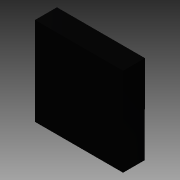
# Autodesk Inventor part: ADP1650
Saved by Autodesk Inventor 2013 (Build 170138000, 138)
## iProperties
Created: 2015-07-04
Part Number: ADP1650
Material: Ogólny
Document SubType Name: Modeling
Designer: terg
Density: 1 g/cm^3
Author: terg
Autodesk Inventor part; units mm, degrees
ref_plane "YZ Plane" through (0, 0, 0) normal (1, 0, 0) x (0, 1, 0)
ref_plane "XZ Plane" through (0, 0, 0) normal (0, 1, 0) x (-1, 0, 0)
ref_plane "XY Plane" through (0, 0, 0) normal (0, 0, 1) x (1, 0, 0)
sketch "Szkic1" plane through (0, 0, 0) normal (0, 1, 0) x (-1, 0, 0)
  line L0 (0, 0) -> (3, 0)
  line L1 (3, 0) -> (3, 3)
  line L2 (3, 3) -> (0, 3)
  line L3 (0, 3) -> (0, 0)
  dimension "d0" = 3
  dimension "d1" = 3
  constraints: 8 end point, 2 parallel, 1 horizontal, 1 perpendicular
  measures "d0" distance of L2.end L1.end
  measures "d1" distance of L1.end L0.end
extrude "Wyciągnięcie proste1" add sketch "Szkic1" along normal blind 0.75
sketch "Szkic2" plane through (0, 0.75, 0) normal (0, 1, 0) x (1, 0, 0)
  line L0 (0, 0) -> (-1.5, 0)
  line L1 (-1.5, 0) -> (-1.5, -1.5)
  line L2 (-1.5, -1.5) -> (0, -1.5)
  line L3 (0, -1.5) -> (0, 0)
  dimension "d4" = 1.5
  dimension "d5" = 1.5
  constraints: 8 end point, 2 parallel, 1 horizontal, 1 perpendicular
  measures "d4" distance of L2.end L1.end
  measures "d5" distance of L1.end L0.end
extrude "Wyciągnięcie proste2" cut sketch "Szkic2" against normal blind 0.01
